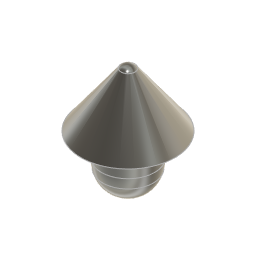
_TopPlug.f9e0ff63-29a4-42b6-9aa4-25f3ffe894e4 (Autodesk Fusion 360 design; units mm, degrees)
Autodesk Fusion 360 part; units mm, degrees
note: some values were not read from the file. Set by a fixed rule: which sketch regions a step uses.
sketch "Sketch1" plane through (0, 0, 0) normal (1, 0, 0) x (0, 1, 0)
  line L0 (0, 0) -> (0, 80)
  line L1 (0, 30) -> (15.5, 30) construction
  line L2 (15.5, 30) -> (16.3627, 41.2147)
  arc A0 (0, 0) -> (15.5, 30) centre (-27.7165, 33.3243) ccw construction
  line L3 (16.5, 43) -> (27, 43)
  line L4 (27, 43) -> (0, 80) construction
  arc A1 (4.039, 74.4651) -> (0, 76.5178) centre (0, 71.5178) ccw
  line L5 (0, 76.5178) -> (-5.7344, 76.5178) construction
  line L6 (0, 12.3924) -> (-9.0357, 12.3924) construction
  arc A2 (0, 12.3924) -> (14.6678, 24.2532) centre (0, 27.3924) ccw
  arc A3 (14.6678, 24.2532) -> (15.5, 30) centre (-27.7165, 33.3243) ccw
  line L7 (4.039, 74.4651) -> (27, 43)
  line L8 (27, 43) -> (9.2494, 55.0378)
  line L9 (8.5592, 54.3371) -> (15.4727, 44.4666)
  line L10 (21.75, 43) -> (0, 63) construction
  arc A4 (16.3627, 41.2147) -> (15.4727, 44.4666) centre (11.3774, 41.5982) ccw
  arc A5 (9.2494, 55.0378) -> (8.5592, 54.3371) centre (8.9688, 54.624) ccw
  point P0 (7, 56.5632)
  dimension "d1" = 80
  dimension "d4" = 30
  dimension "d5" = 27
  dimension "d6" = 15.5
  dimension "d7" = 16.5
  dimension "d8" = 13
  dimension "d9" = 5
  dimension "d10" = 15
  dimension "d12" = 17
  dimension "d13" = 7
  dimension "d14" = 5
  dimension "d15" = 0.5
  constraint coincident L0.start A0.start
  constraint vertical L0
  constraint coincident L0 L1.start
  constraint perpendicular L0 L1
  constraint tangent L2 A0
  constraint horizontal L3
  constraint tangent L4 A1
  constraint coincident L0 A1.end
  constraint coincident L4 A1.start
  constraint perpendicular L0 L5
  constraint tangent A1 L5
  constraint coincident L0 L6.start
  constraint perpendicular L0 L6
  constraint tangent L6 A2
  constraint coincident A0 A2.end
  constraint tangent A0 A2
  constraint coincident A0.centre A3.centre
  constraint midpoint L3 L10.start
  constraint coincident L0 L10.end
  constraint coincident P0 L10
  constraint coincident L3.start L9
  constraint coincident L3.start L2
  constraint tangent L9 A4
  constraint tangent L2 A4
  constraint coincident P0 L9
  constraint coincident P0 L8
  constraint tangent L9 A5
  constraint tangent L8 A5
  measures "d1" distance of L0.start L0.end
  measures "d4" distance of L0.start L1
  measures "d5" distance of L0 L3.end
  measures "d6" distance of L0 L1.end
  measures "d7" distance of L0 L3.start
  measures "d8" distance of L1.end L3
  measures "d9" radius of A1
  measures "d10" radius of A2
  measures "d12" distance of L0.end L10.end
  measures "d13" distance of L0 P0
  measures "d14" radius of A4
  measures "d15" radius of A5
revolve "Revolve1" add sketch "Sketch1" angle 360 about axis through (0, 0, 0) along (0, 0, 1)
